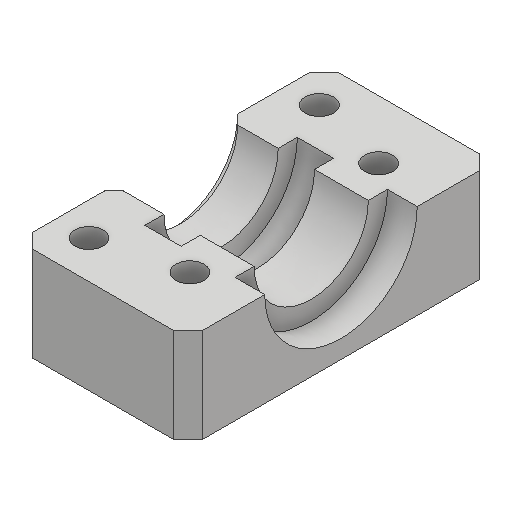
# Autodesk Inventor part: 3DP_ABS_E3D_V6_Mount
Saved by Autodesk Inventor 2026.1 (Build 301233000, 233)
## iProperties
Created: 2016-06-18
Part Number: 3DP_ABS_E3D_V6_Mount
Material: Ogólny
Document SubType Name: Modeling
Designer: Andrzej
Density: 1 g/cm^3
Appearance: Domyślna
Mass: 4.98789 g
Surface Area: 30.2543 cm^2
Volume: 4.98789 cm^3
Author: Andrzej
Autodesk Inventor part; units mm, degrees
ref_plane "YZ Plane" through (0, 0, 0) normal (1, 0, 0) x (0, 1, 0)
ref_plane "XZ Plane" through (0, 0, 0) normal (0, 1, 0) x (-1, 0, 0)
ref_plane "XY Plane" through (0, 0, 0) normal (0, 0, 1) x (1, 0, 0)
sketch "Szkic1" plane through (0, 0, 0) normal (0, 0, 1) x (1, 0, 0)
  line L0 (-10.699, 18.8462) -> (5.301, 18.8462)
  line L1 (5.301, 18.8462) -> (5.301, -13.5538)
  line L2 (5.301, -13.5538) -> (-10.699, -13.5538)
  line L3 (-10.699, -13.5538) -> (-10.699, 18.8462)
  point P0 (0, 0)
  dimension "d0" = 16
  dimension "d1" = 32.4
  constraints: 8 end point, 2 parallel, 1 horizontal, 1 perpendicular
  measures "d0" distance of L1.end L2.end
  measures "d1" distance of L0.end L1.end
extrude "Wyciągnięcie proste1" add sketch "Szkic1" along normal blind 10
sketch "Szkic2" plane through (-10.699, -13.5538, 0) normal (-1, 0, 0) x (0, 0, 1)
  line L0 (0, 0) -> (0, 32.4) projected
  line L1 (0, 0) -> (10, 0) projected
  line L2 (10, 32.4) -> (10, 0) projected
  line L3 (0, 32.4) -> (10, 32.4) projected
  line L4 (10, 32.4) -> (10, 0) projected
  circle A0 centre (10, 16.2) radius 6.05
  point P0 (0, 13.5538)
  dimension "d4" = 32.4
  dimension "d5" = 16.2
  dimension "d6" = 12.1
  constraints: 1 centre point, 1 coincident, 1 midpoint
  measures "d4" distance of L2.start L1.end
  measures "d5" distance from line of L3 point (10, 16.2)
  measures "d6" diameter of A0
extrude "Wyciągnięcie proste2" cut sketch "Szkic2" against normal blind 13 contours A0 L2 | L2 A0
sketch "Szkic3" plane through (-10.699, -13.5538, 0) normal (-1, 0, 0) x (0, 0, 1)
  arc A0 (10, 22.25) -> (10, 10.15) centre (10, 16.2) ccw projected
  line L0 (10, 32.4) -> (10, 22.25) projected
  line L1 (0, 32.4) -> (10, 32.4) projected
  line L2 (0, 0) -> (0, 32.4) projected
  line L3 (0, 0) -> (10, 0) projected
  line L4 (10, 10.15) -> (10, 0) projected
  arc A1 (10, 24.275) -> (10, 8.125) centre (10, 16.2) ccw
  point P0 (0, 13.5538)
  dimension "d9" = 16.15
  constraints: 2 point on circle, 2 point on line, 1 centre point, 1 coincident
  measures "d9" diameter of A1
extrude "Wyciągnięcie proste3" cut sketch "Szkic3" against normal blind 7.15 contours A0 L4 A1 L0
extrude "Wyciągnięcie proste4" add sketch "Szkic3" against normal blind 3.3 contours A0 L4 A1 L0
sketch "Szkic6" plane through (5.301, -13.5538, 0) normal (1, 0, 0) x (0, 0, -1)
  arc A0 (-10, 8.125) -> (-10, 24.275) centre (-10, 16.2) ccw projected
  line L0 (0, 32.4) -> (0, 0) projected
  line L1 (0, 32.4) -> (-10, 32.4) projected
  line L2 (-10, 0) -> (-10, 32.4) projected
  line L3 (0, 0) -> (-10, 0) projected
  arc A1 (-10, 8.125) -> (-10, 24.275) centre (-10, 16.2) ccw
  point P0 (0, 13.5538)
  constraints: 2 point on circle, 2 point on line, 1 centre point, 1 coincident, 1 concentric
extrude "Wyciągnięcie proste5" cut sketch "Szkic6" against normal blind 3.15 contours L2 A0
sketch "Szkic7" plane through (0, 0, 10) normal (0, 0, 1) x (1, 0, 0)
  line L0 (5.301, -5.4288) -> (2.151, -5.4288) projected
  line L1 (2.151, -5.4288) -> (2.151, -3.4038) projected
  line L2 (2.151, -3.4038) -> (-3.549, -3.4038) projected
  line L3 (-3.549, -3.4038) -> (-3.549, -5.4288) projected
  line L4 (-3.549, -5.4288) -> (-7.399, -5.4288) projected
  line L5 (-7.399, -3.4038) -> (-7.399, -5.4288) projected
  line L6 (-10.699, -3.4038) -> (-7.399, -3.4038) projected
  line L7 (-10.699, -3.4038) -> (-10.699, -13.5538) projected
  line L8 (-10.699, -13.5538) -> (5.301, -13.5538) projected
  line L9 (5.301, -13.5538) -> (5.301, -5.4288) projected
  line L10 (2.151, 10.7212) -> (5.301, 10.7212) projected
  line L11 (5.301, 10.7212) -> (5.301, 18.8462) projected
  line L12 (5.301, 18.8462) -> (-10.699, 18.8462) projected
  line L13 (-10.699, 18.8462) -> (-10.699, 8.6962) projected
  line L14 (-10.699, 8.6962) -> (-7.399, 8.6962) projected
  line L15 (-7.399, 10.7212) -> (-7.399, 8.6962) projected
  line L16 (-7.399, 10.7212) -> (-3.549, 10.7212) projected
  line L17 (-3.549, 10.7212) -> (-3.549, 8.6962) projected
  line L18 (-3.549, 8.6962) -> (2.151, 8.6962) projected
  line L19 (2.151, 8.6962) -> (2.151, 10.7212) projected
  point P0 (0, 0)
  point P1 (-0.699, -7.3538)
  point P2 (-0.699, 12.6462)
  dimension "d46" = 20
  dimension "d47" = 32.4
  dimension "d48" = 6.2
  dimension "d49" = 6.2
  dimension "d50" = 5.7
  dimension "d96" = 10
  dimension "d97" = 10
  measures "d46" distance of point (-0.699, 12.646) point (-0.699, -7.354)
  measures "d47" distance between parallel lines of L12 L8
  measures "d48" distance from line of L8 point (-0.699, -7.354)
  measures "d49" distance from line of L12 point (-0.699, 12.646)
  measures "d50" distance between parallel lines of L1 L3
  measures "d96" distance from line of L7 point (-0.699, -7.354)
  measures "d97" distance from line of L13 point (-0.699, 12.646)
hole "Otwór3" at (-0.699, -7.3538, 10) at (-0.699, 12.6462, 10) direction (0, 0, -1) diameter 3 end through all
chamfer "Faza4" distance 1.5 angle 45 2 edges at (5.301, -13.5538, 5) (5.301, 18.8462, 5)
sketch "Szkic9" plane through (-10.699, -13.5538, 0) normal (-1, 0, 0) x (0, 0, 1)
  line L0 (10, 32.4) -> (10, 22.25) projected
  line L1 (0, 32.4) -> (10, 32.4) projected
  line L2 (0, 0) -> (0, 32.4) projected
  line L3 (0, 0) -> (10, 0) projected
  line L4 (10, 10.15) -> (10, 0) projected
  arc A0 (10, 22.25) -> (10, 10.15) centre (10, 16.2) ccw projected
  point P0 (0, 13.5538)
extrude "Wyciągnięcie proste7" add sketch "Szkic9" along normal blind 2
chamfer "Faza8" distance 1.5 angle 45 2 edges at (-12.699, -13.5538, 5) (-12.699, 18.8462, 5)
chamfer "Faza9" distance 1 angle 45 1 edges at (-12.699, 2.6462, 3.95)
sketch "Szkic10" plane through (0, 0, 10) normal (0, 0, 1) x (1, 0, 0)
  circle A0 centre (-0.699, -7.3538) radius 1.5 projected
  line L0 (-12.699, -4.4038) -> (-11.699, -3.4038) projected
  line L1 (-12.699, -12.0538) -> (-12.699, -4.4038) projected
  line L2 (-11.199, -13.5538) -> (-12.699, -12.0538) projected
  line L3 (3.801, -13.5538) -> (-11.199, -13.5538) projected
  line L4 (5.301, -12.0538) -> (3.801, -13.5538) projected
  line L5 (5.301, -12.0538) -> (5.301, -5.4288) projected
  line L6 (5.301, -5.4288) -> (2.151, -5.4288) projected
  line L7 (2.151, -5.4288) -> (2.151, -3.4038) projected
  line L8 (2.151, -3.4038) -> (-3.549, -3.4038) projected
  line L9 (-3.549, -3.4038) -> (-3.549, -5.4288) projected
  line L10 (-3.549, -5.4288) -> (-7.399, -5.4288) projected
  line L11 (-7.399, -3.4038) -> (-7.399, -5.4288) projected
  line L12 (-11.699, -3.4038) -> (-7.399, -3.4038) projected
  line L13 (-11.699, 8.6962) -> (-12.699, 9.6962) projected
  line L14 (-7.399, 8.6962) -> (-11.699, 8.6962) projected
  line L15 (-7.399, 10.7212) -> (-7.399, 8.6962) projected
  line L16 (-7.399, 10.7212) -> (-3.549, 10.7212) projected
  line L17 (-3.549, 10.7212) -> (-3.549, 8.6962) projected
  line L18 (-3.549, 8.6962) -> (2.151, 8.6962) projected
  line L19 (2.151, 8.6962) -> (2.151, 10.7212) projected
  line L20 (2.151, 10.7212) -> (5.301, 10.7212) projected
  line L21 (5.301, 10.7212) -> (5.301, 17.3462) projected
  line L22 (3.801, 18.8462) -> (5.301, 17.3462) projected
  line L23 (3.801, 18.8462) -> (-11.199, 18.8462) projected
  line L24 (-12.699, 17.3462) -> (-11.199, 18.8462) projected
  line L25 (-12.699, 9.6962) -> (-12.699, 17.3462) projected
  circle A1 centre (-0.699, 12.6462) radius 1.5 projected
  point P0 (0, 0)
  point P1 (-9.199, -9.5538)
  point P2 (-9.199, 14.8462)
  dimension "d106" = 4
  dimension "d107" = 4
  dimension "d108" = 3.5
  dimension "d109" = 3.5
  measures "d106" distance from line of L3 point (-9.199, -9.554)
  measures "d107" distance from line of L23 point (-9.199, 14.846)
  measures "d108" distance from line of L1 point (-9.199, -9.554)
  measures "d109" distance from line of L25 point (-9.199, 14.846)
hole "Otwór4" at (-9.199, -9.5538, 10) at (-9.199, 14.8462, 10) direction (0, 0, -1) diameter 3 end through all
equation "\"d5\" = 0.5 * d4"
equation "\"d48\" = -0.5 * d46 + 0.5 * d47"
